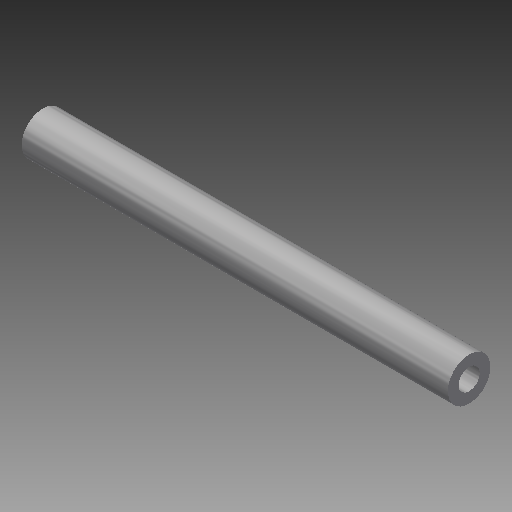
# Autodesk Inventor part: Shaft
Saved by Autodesk Inventor 2019.4 (Build 234330000, 330)
## iProperties
Created: 2020-01-01
Part Number: Shaft
Material: Steel
Document SubType Name: Modeling
Designer: Mark
Density: 7.85 g/cm^3
Appearance: Steel
Mass: 50.2503 g
Surface Area: 41.5319 cm^2
Volume: 6.40131 cm^3
CustomPartVersion: 1
Length: 100.000 mm
Author: Mark
Autodesk Inventor part; units mm, degrees
ref_plane "Start Plane" through (0, 0, 0) normal (1, 0, 0) x (0, 1, 0)
ref_plane "XZ Plane" through (0, 0, 0) normal (0, 1, 0) x (-1, 0, 0)
ref_plane "XY Plane" through (0, 0, 0) normal (0, 0, 1) x (1, 0, 0)
sketch "Main Sketch" plane through (0, 0, 0) normal (0, 0, 1) x (1, 0, 0)
  line L0 (0, 0) -> (100, 0)
  line L1 (0, 2.5) -> (0, 5)
  line L2 (100, 5) -> (100, 2.5)
  line L3 (0, 5) -> (100, 5)
  line L4 (20, 2.5) -> (20, 0)
  line L5 (0, 2.5) -> (20, 2.5)
  line L6 (80, 2.5) -> (80, 0)
  line L7 (100, 2.5) -> (80, 2.5)
  line L8 (20, 0) -> (80, 0)
  dimension "d3" = 10
  dimension "d4" = 5
  dimension "d5" = 5
  constraints: 18 end point, 4 horizontal, 4 vertical
  measures "d3" diameter of L3 L0
  measures "d4" diameter of L5 L0
  measures "d5" diameter of L7 L0
revolve "Revolution1" add sketch "Main Sketch" angle 360 about axis through (0, 0, 0) along (1, 0, 0)
equation "\"Length\" = 100"
body "Solid1"
